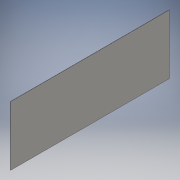
# Autodesk Inventor part: Opening flap_Side2Side Motion
Saved by Autodesk Inventor 2016 (Build 200138000, 138)
## iProperties
Created: 2016-04-02
Part Number: Opening flap_Side2Side Motion
Material: Generic
Document SubType Name: Modeling
Designer: aoben3
Density: 1 g/cm^3
Appearance: Default
Author: aoben3
Autodesk Inventor part; units mm, degrees
ref_plane "YZ Plane" through (0, 0, 0) normal (1, 0, 0) x (0, 1, 0)
ref_plane "XZ Plane" through (0, 0, 0) normal (0, 1, 0) x (-1, 0, 0)
ref_plane "XY Plane" through (0, 0, 0) normal (0, 0, 1) x (1, 0, 0)
sketch "Sketch1" plane through (0, 0, 0) normal (1, 0, 0) x (0, 1, 0)
  line L0 (57.15, 152.4) -> (-57.15, 152.4)
  line L1 (-57.15, 152.4) -> (-57.15, -152.4)
  line L2 (-57.15, -152.4) -> (57.15, -152.4)
  line L3 (57.15, -152.4) -> (57.15, 152.4)
  line L4 (57.15, 152.4) -> (-57.15, -152.4) construction
  line L5 (-57.15, 152.4) -> (57.15, -152.4) construction
  point P0 (0, 0)
  dimension "d0" = 114.3
  dimension "d1" = 304.8
  constraints: 12 end point, 2 midpoint, 2 parallel, 1 horizontal, 1 perpendicular
  measures "d0" distance of L1.end L2.end
  measures "d1" distance of L2.end L0.start
extrude "Extrusion1" add sketch "Sketch1" along normal blind 0.3969
body "Solid1"
